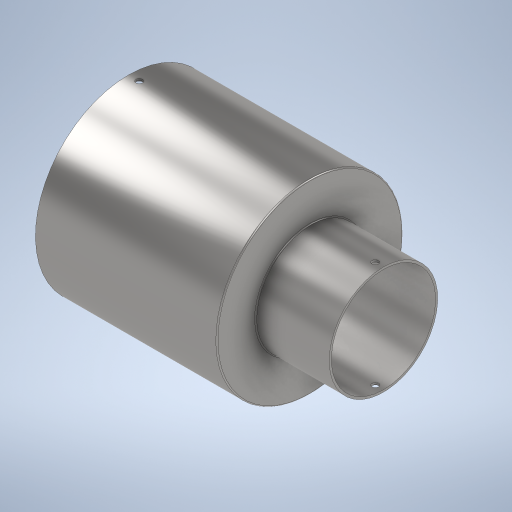
# Autodesk Inventor part: new outer wall
Saved by Autodesk Inventor 2023 (Build 270158000, 158)
## iProperties
Created: 2022-07-21
Part Number: new outer wall
Material: Stainless Steel
Document SubType Name: Modeling
Designer: station
Density: 8 g/cm^3
Appearance: Semi-Polished
Author: station
Autodesk Inventor part; units mm, degrees
ref_plane "YZ Plane" through (0, 0, 0) normal (1, 0, 0) x (0, 1, 0)
ref_plane "XY Plane" through (0, 0, 0) normal (0, 0, 1) x (1, 0, 0)
sketch "Sketch1" plane through (0, 0, 0) normal (0, 0, 1) x (1, 0, 0)
  arc A0 (180.1312, 21.4516) -> (182.1847, 21.7676) centre (180.1312, 28.2803) ccw
  arc A1 (166.724, 25.044) -> (180.1312, 21.4516) centre (180.1312, 48.266) ccw
  line L0 (123.3912, 50.0622) -> (166.724, 25.044)
  arc A2 (123.3912, 50.0622) -> (30.0219, 75.0805) centre (30.0219, -111.6581) ccw
  line L1 (0, 75.0805) -> (30.0219, 75.0805)
  line L2 (0, 3.5755) -> (0, 203.5755) construction
  line L3 (0, 3.5755) -> (319.1694, 3.5755)
  line L4 (0, 77.0805) -> (30.0219, 77.0805)
  arc A3 (124.3912, 51.7943) -> (30.0219, 77.0805) centre (30.0219, -111.6581) ccw
  line L5 (124.3912, 51.7943) -> (167.724, 26.7761)
  arc A4 (167.724, 26.7761) -> (180.1312, 23.4516) centre (180.1312, 48.266) ccw
  arc A5 (180.1312, 23.4516) -> (181.5842, 23.6753) centre (180.1312, 28.2803) ccw
  line L6 (182.1847, 21.7676) -> (237.115, 39.0871)
  line L7 (236.5136, 40.9945) -> (181.5833, 23.6751)
  arc A6 (180.1312, 23.4516) -> (181.5833, 23.6751) centre (180.1312, 28.2803) ccw
  line L8 (236.5136, 40.9945) -> (237.115, 39.0871)
  line L9 (0, 88.1805) -> (30.0219, 88.1805)
  line L10 (166.724, 25.044) -> (166.724, -4.6444)
  line L11 (30.0219, 88.1805) -> (165.724, 88.1805)
  line L12 (237.115, 39.0871) -> (233.0254, 52.0576)
  line L13 (236.5136, 40.9945) -> (233.0254, 52.0576)
  line L14 (233.0254, 52.0576) -> (144.4694, 24.136)
  line L15 (233.0254, 52.0576) -> (237.115, 52.0576)
  line L16 (233.0254, 52.0576) -> (167.724, 52.0576)
  line L17 (167.724, 90.1805) -> (30.0219, 90.1805)
  line L18 (30.0219, 90.1805) -> (0, 90.1805)
  line L19 (233.0254, 54.0576) -> (169.724, 54.0576)
  line L20 (168.724, 25.044) -> (168.724, 31.7835)
  line L21 (168.724, 55.0576) -> (168.724, 89.1805)
  line L22 (166.724, 25.044) -> (166.724, 31.1529)
  line L23 (166.724, 53.0576) -> (166.724, 87.1805)
  arc A7 (166.724, 87.1805) -> (165.724, 88.1805) centre (165.724, 87.1805) ccw
  arc A8 (168.724, 89.1805) -> (167.724, 90.1805) centre (167.724, 89.1805) ccw
  arc A9 (168.724, 55.0576) -> (169.724, 54.0576) centre (169.724, 55.0576) ccw
  arc A10 (166.724, 53.0576) -> (167.724, 52.0576) centre (167.724, 53.0576) ccw
  line L24 (0, 88.1805) -> (0, 90.1805)
  line L25 (237.115, 52.0576) -> (237.115, 54.0576)
  line L26 (233.0254, 54.0576) -> (237.115, 54.0576)
  dimension "d48" = 200
  dimension "d49" = 30.0219
  dimension "d50" = 186.7386
  dimension "d51" = 0
  dimension "d52" = 0
  dimension "d53" = 0
  dimension "d54" = 71.505
  dimension "d55" = 2
  dimension "d56" = 2
  dimension "d57" = 2
  dimension "d58" = 2
  dimension "d59" = 2
  dimension "d60" = 17.5
  dimension "d61" = 54.9303
  dimension "d62" = 2
  dimension "d63" = 11.1
  dimension "d66" = 11.6
  dimension "d67" = 17.5
  dimension "d68" = 2
  dimension "d69" = 2
  dimension "d70" = 1
  dimension "d71" = 1
  dimension "d72" = 1
  dimension "d73" = 1
  constraints: 54 end point, 22 point on circle, 11 centre point, 9 tangent, 4 horizontal, 4 parallel, 4 vertical, 2 point on line, 1 collinear, 1 perpendicular, 2 other
  measures "d48" distance of L2.start L2.end
  measures "d49" distance of L1.start L1.end
  measures "d50" radius of A2
  measures "d51" distance from line of L1.start L2
  measures "d52" distance of A2.end L1.end
  measures "d53" distance of L0.start A2.start
  measures "d54" distance between parallel lines of L3 L1
  measures "d55" distance between parallel lines of L1 L4
  measures "d56" radial gap between concentric circles of A2 A3
  measures "d57" distance between parallel lines of L0 L5
  measures "d58" radial gap between concentric circles of A1 A4
  measures "d59" radial gap between concentric circles of A0 A5
  measures "d60" angle of L3 L6
  measures "d61" horizontal distance of L6.start L6.end
  measures "d62" distance between parallel lines of L6 L7
  measures "d63" distance between parallel lines of L4 L9
  measures "d66" distance of L12.end L7.start
  measures "d67" angle of L3 L14
  measures "d68" distance between parallel lines of L11 L17
  measures "d69" distance between parallel lines of L16 L19
  measures "d70" radius of A7
  measures "d71" radius of A8
  measures "d72" radius of A9
  measures "d73" radius of A10
revolve "Revolution3" add sketch "Sketch1" angle 360 about axis through (0, 3.5755, 0) along (1, 0, 0) contours L16 A10 L23 A7 L11 L9 L24 L18 L17 A8 L21 A9 L19 L26 L25 L15
ref_plane "Work Plane1" through (0, 100, 0) normal (0, 1, 0) x (-1, 0, 0)
sketch "Sketch3" plane through (0, 100, 0) normal (0, 1, 0) x (-1, 0, 0)
  line L0 (0, 0) -> (-10, 0)
  circle A0 centre (-10, 0) radius 3
  dimension "d39" = 10
  dimension "d40" = 6
  constraints: 2 end point, 1 centre point, 1 coincident, 1 horizontal
  measures "d39" distance of L0.start L0.end
  measures "d40" diameter of A0
extrude "Extrusion2" cut sketch "Sketch3" against normal through all
thread "Thread2" size "M6x1" class "6H" standard "ANSI Metric M Profile" full length
thread "Thread3" size "M6x1" class "6H" standard "ANSI Metric M Profile" full length
ref_plane "Work Plane2" through (0, 59.5, 0) normal (0, 1, 0) x (-1, 0, 0)
sketch "Sketch4" plane through (0, 59.5, 0) normal (0, 1, 0) x (-1, 0, 0)
  line L0 (-237.115, 50.4822) -> (-237.115, -50.4822) projected
  line L1 (-237.115, 0) -> (-229.514, 0)
  circle A0 centre (-229.514, 0) radius 3
  point P0 (0, 0)
  dimension "d79" = 7.601
  dimension "d80" = 6
  constraints: 2 end point, 1 centre point, 1 coincident, 1 horizontal, 1 midpoint
  measures "d79" distance of L1.start L1.end
  measures "d80" diameter of A0
extrude "Extrusion3" cut sketch "Sketch4" against normal through all
thread "Thread4" size "M6x1" class "6H" standard "ANSI Metric M Profile" full length
thread "Thread5" size "M6x1" class "6H" standard "ANSI Metric M Profile" full length
body "Solid3"
